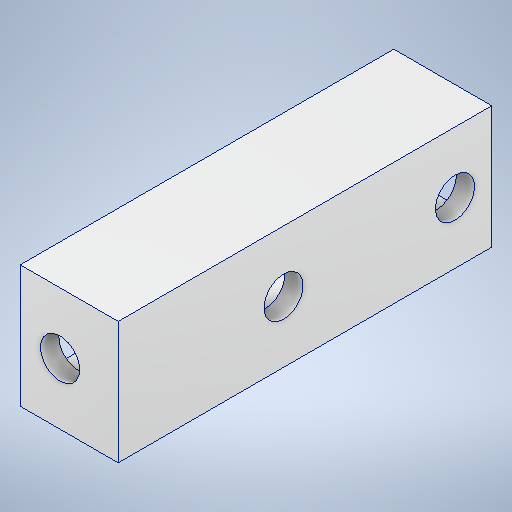
# Autodesk Inventor part: lift_tab_bracket
Saved by Autodesk Inventor 2025 (Build 290162000, 162)
## iProperties
Created: 2024-04-25
Part Number: lift_tab_bracket
Material: Hliník 6061
Document SubType Name: Modeling
Designer: rader
Density: 2.7 g/cm^3
Appearance: Hliník – plochý
Author: rader
Autodesk Inventor part; units mm, degrees
ref_plane "YZ Plane" through (0, 0, 0) normal (1, 0, 0) x (0, 1, 0)
ref_plane "XZ Plane" through (0, 0, 0) normal (0, 1, 0) x (-1, 0, 0)
ref_plane "XY Plane" through (0, 0, 0) normal (0, 0, 1) x (1, 0, 0)
sketch "Náčrt1" plane through (0, 0, 0) normal (0, 1, 0) x (-1, 0, 0)
  line L0 (0, -2) -> (0, 12) projected
  line L1 (-1.6, 0) -> (9.6, 0) projected
  line L2 (8, 10) -> (0, 10)
  line L3 (0, 10) -> (0, 0)
  line L4 (0, 0) -> (8, 0)
  line L5 (8, 0) -> (8, 10)
  line L6 (8, 8.5) -> (1.5, 8.5)
  line L7 (1.5, 8.5) -> (1.5, 1.5)
  line L8 (1.5, 1.5) -> (8, 1.5)
  line L9 (8, 1.5) -> (8, 8.5)
  point P0 (0, 0)
  point P1 (0, 10)
  dimension "d0" = 8
  dimension "d1" = 10
  dimension "d2" = 6.5
  dimension "d3" = 7
  dimension "d4" = 1.5
  constraints: 16 end point, 4 parallel, 2 collinear, 2 horizontal, 2 perpendicular, 1 point on line
  measures "d0" distance of L4.end L3.end
  measures "d1" distance of L3.end L2.end
  measures "d2" distance of L8.end L7.end
  measures "d3" distance of L7.end L6.end
  measures "d4" distance between parallel lines of L4 L8
extrude "Vysunutí1" add sketch "Náčrt1" along normal mid plane 29 contours L0 L2 L5 L6 L7 L8 L1
sketch "Náčrt2" plane through (0, -14.5, 0) normal (0, -1, 0) x (1, 0, 0)
  line L0 (-8, 8.5) -> (-1.5, 8.5) projected
  line L1 (-1.5, 8.5) -> (-1.5, 1.5) projected
  line L2 (-1.5, 1.5) -> (-8, 1.5) projected
  line L3 (-8, 1.5) -> (-8, 0) projected
  line L4 (-8, 0) -> (0, 0) projected
  line L5 (0, 0) -> (0, 10) projected
  line L6 (0, 10) -> (-8, 10) projected
  line L7 (-8, 10) -> (-8, 8.5) projected
  line L8 (-8, 10) -> (0, 10)
  line L9 (0, 10) -> (0, 0)
  line L10 (0, 0) -> (-8, 0)
  line L11 (-8, 0) -> (-8, 10)
  constraints: 8 end point, 2 parallel, 1 horizontal, 1 perpendicular
extrude "Vysunutí2" add sketch "Náčrt2" along normal blind 1.5
sketch "Náčrt3" plane through (0, -14.5, 0) normal (0, 1, 0) x (1, 0, 0)
  line L0 (-8, -8.5) -> (-1.5, -8.5) projected
  line L1 (-1.5, -8.5) -> (-1.5, -1.5) projected
  line L2 (-1.5, -1.5) -> (-8, -1.5) projected
  line L3 (-8, -8.5) -> (-8, -1.5) projected
  point P0 (0, 0)
  point P1 (-4.75, -5)
  dimension "d9" = 3.25
  dimension "d10" = 3.5
  measures "d9" distance from line of L3 point (-4.75, -5)
  measures "d10" distance from line of L0 point (-4.75, -5)
hole "Díra1" at (-4.75, -14.5, 5) direction (0, -1, 0) diameter 3.2 end through all
sketch "Náčrt4" plane through (-1.5, 14.5, 1.5) normal (-1, 0, 0) x (0, 0, 1)
  line L0 (0, 0) -> (7, 0) projected
  line L1 (7, 0) -> (7, -29) projected
  line L2 (0, 0) -> (7, 0) projected
  line L3 (0, -29) -> (0, 0) projected
  line L4 (7, -29) -> (0, -29) projected
  point P0 (-1.5, -14.5)
  point P1 (3.5, -3)
  point P2 (3.5, -17)
  point P3 (3.5, 0)
  dimension "d18" = 3
  dimension "d19" = 14
  dimension "d20" = 3.5
  dimension "d21" = 3.5
  constraints: 1 midpoint
  measures "d18" distance of point (3.5, 0) point (3.5, -3)
  measures "d19" distance of point (3.5, -3) point (3.5, -17)
  measures "d20" distance from line of L3 point (3.5, -3)
  measures "d21" distance from line of L3 point (3.5, -17)
hole "Díra2" at (-1.5, 11.5, 5) at (-1.5, -2.5, 5) direction (1, 0, 0) diameter 3.2 end through all
